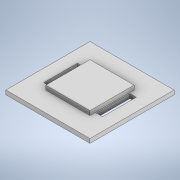
# Autodesk Inventor part: Test_Button_Backboard
Saved by Autodesk Inventor 2021 (Build 250183000, 183)
## iProperties
Created: 2020-06-01
Part Number: Test_Button_Backboard
Material: Generic
Document SubType Name: Modeling
Designer: ameli
Density: 1 g/cm^3
Appearance: Default
Author: ameli
Autodesk Inventor part; units mm, degrees
ref_plane "YZ Plane" through (0, 0, 0) normal (1, 0, 0) x (0, 1, 0)
ref_plane "XZ Plane" through (0, 0, 0) normal (0, 1, 0) x (-1, 0, 0)
ref_plane "XY Plane" through (0, 0, 0) normal (0, 0, 1) x (1, 0, 0)
sketch "Sketch1" plane through (0, 0, 0) normal (0, 1, 0) x (-1, 0, 0)
  line L0 (0, 0) -> (20, 0)
  line L1 (20, 0) -> (20, -20)
  line L2 (20, -20) -> (0, -20)
  line L3 (0, -20) -> (0, 0)
  dimension "d0" = 20
  dimension "d1" = 20
  constraints: 8 end point, 2 parallel, 1 horizontal, 1 perpendicular
  measures "d0" distance of L0.end L1.end
  measures "d1" distance of L1.end L2.end
extrude "Extrusion1" add sketch "Sketch1" along normal blind 1
sketch "Sketch2" plane through (0, 1, 0) normal (0, 1, 0) x (1, 0, 0)
  line L0 (-15.5, 4.5) -> (-4.5, 4.5) construction
  line L1 (-4.5, 4.5) -> (-4.5, 15.5) construction
  line L2 (-4.5, 15.5) -> (-15.5, 15.5) construction
  line L3 (-15.5, 15.5) -> (-15.5, 4.5) construction
  line L4 (0, 0) -> (0, 20) projected
  line L5 (0, 20) -> (-20, 20) projected
  line L6 (-15.25, 15.25) -> (-4.75, 15.25)
  line L7 (-4.75, 15.25) -> (-4.75, 4.75)
  line L8 (-4.75, 4.75) -> (-15.25, 4.75)
  line L9 (-15.25, 4.75) -> (-15.25, 15.25)
  dimension "d4" = 11
  dimension "d5" = 11
  dimension "d6" = 4.5
  dimension "d7" = 4.5
  dimension "d20" = 0.25
  constraints: 16 end point, 4 parallel, 2 perpendicular, 1 horizontal, 3 other
  measures "d4" distance of L2.end L0.start
  measures "d5" distance of L1.end L2.end
  measures "d6" distance between parallel lines of L4 L1
  measures "d7" distance between parallel lines of L5 L2
  measures "d20" distance between parallel lines of L2 L6
extrude "Extrusion2" add sketch "Sketch2" along normal blind 1
sketch "Sketch3" plane through (0, 1, 0) normal (0, 1, 0) x (1, 0, 0)
  line L0 (-4.5, 14) -> (-3, 14)
  line L1 (-3, 14) -> (-3, 6)
  line L2 (-3, 6) -> (-4.5, 6)
  line L3 (-4.5, 6) -> (-4.5, 14)
  line L4 (-4.5, 4.5) -> (-4.5, 15.5) projected
  line L5 (-4.5, 15.5) -> (-15.5, 15.5) projected
  line L6 (-15.5, 14) -> (-17, 14)
  line L7 (-17, 14) -> (-17, 6)
  line L8 (-17, 6) -> (-15.5, 6)
  line L9 (-15.5, 6) -> (-15.5, 14)
  line L10 (-15.5, 15.5) -> (-15.5, 4.5) projected
  line L11 (-15.5, 4.5) -> (-4.5, 4.5) projected
  point P0 (0, 0)
  dimension "d10" = 8
  dimension "d11" = 1.5
  dimension "d12" = 0
  dimension "d13" = 1.5
  dimension "d14" = 8
  dimension "d15" = 1.5
  dimension "d16" = 0
  dimension "d17" = 1.5
  constraints: 16 end point, 4 parallel, 2 horizontal, 2 perpendicular
  measures "d10" distance of L0.end L1.end
  measures "d11" distance of L1.end L2.end
  measures "d12" distance between parallel lines of L4 L3
  measures "d13" distance between parallel lines of L5 L0
  measures "d14" distance of L8.end L6.start
  measures "d15" distance of L6.start L6.end
  measures "d16" distance between parallel lines of L10 L9
  measures "d17" distance between parallel lines of L11 L8
extrude "Extrusion3" cut sketch "Sketch3" against normal through all contours L0 L1 L2 L3 | L9 L8 L7 L6
body "Solid1"
